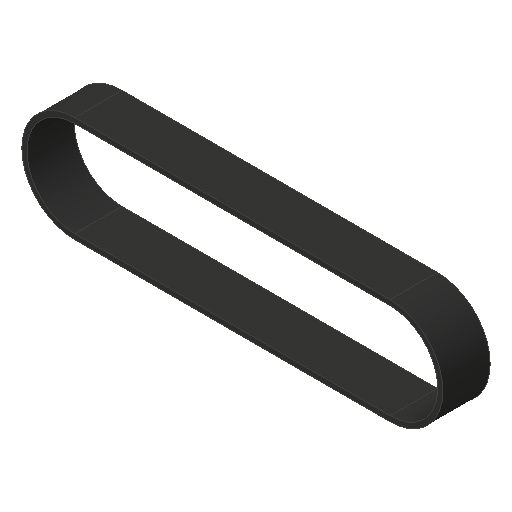
# Autodesk Inventor part: COTS_GENERIC_GT2_Timing_belt_6mm_closed_loop_stepper
Saved by Autodesk Inventor 2026.1 (Build 301233000, 233)
## iProperties
Created: 2018-06-17
Part Number: COTS_GENERIC_GT2_Timing_belt_6mm_closed_loop_stepper
Material: Generic
Document SubType Name: Modeling
Designer: Andrzej
Density: 1 g/cm^3
Appearance: Rubber - Black
Author: Andrzej
Autodesk Inventor part; units mm, degrees
ref_plane "YZ Plane" through (0, 0, 0) normal (1, 0, 0) x (0, 1, 0)
ref_plane "XZ Plane" through (0, 0, 0) normal (0, 1, 0) x (-1, 0, 0)
ref_plane "XY Plane" through (0, 0, 0) normal (0, 0, 1) x (1, 0, 0)
sketch "Sketch1" plane through (0, 0, 0) normal (0, 0, 1) x (1, 0, 0)
  line L0 (-12.0437, 0) -> (27.9563, 0) construction
  line L1 (-12.0437, -6.05) -> (27.9563, -6.05)
  line L2 (27.9563, 6.05) -> (-12.0437, 6.05)
  arc A0 (-12.0437, 6.05) -> (-12.0437, -6.05) centre (-12.0437, 0) ccw
  arc A1 (27.9563, -6.05) -> (27.9563, 6.05) centre (27.9563, 0) ccw
  line L3 (-12.0437, -6.7) -> (27.9563, -6.7)
  arc A2 (27.9563, -6.7) -> (27.9563, 6.7) centre (27.9563, 0) ccw
  line L4 (27.9563, 6.7) -> (-12.0437, 6.7)
  arc A3 (-12.0437, 6.7) -> (-12.0437, -6.7) centre (-12.0437, 0) ccw
  point P0 (0, 0)
  point P1 (7.9563, 0)
  dimension "d0" = 40
  dimension "d1" = 12.1
  dimension "d2" = 0.65
  constraints: 12 end point, 8 point on circle, 4 centre point, 4 tangent, 2 parallel, 1 horizontal, 1 midpoint, 3 other
  measures "d0" distance of L0.start L0.end
  measures "d1" diameter of A1
  measures "d2" radial gap between concentric circles of A0 A3
extrude "Extrusion1" add sketch "Sketch1" along normal blind 6
body "Solid1"
